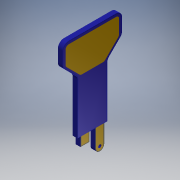
# Autodesk Inventor part: KeyerPaddle
Saved by Autodesk Inventor 2016 (Build 200138000, 138)
## iProperties
Created: 2016-06-11
Part Number: KeyerPaddle
Material: Generic
Document SubType Name: Modeling
Designer: Tyler
Density: 1 g/cm^3
Appearance: Default
Author: Tyler
Autodesk Inventor part; units mm, degrees
ref_plane "YZ Plane" through (0, 0, 0) normal (1, 0, 0) x (0, 1, 0)
ref_plane "XZ Plane" through (0, 0, 0) normal (0, 1, 0) x (-1, 0, 0)
ref_plane "XY Plane" through (0, 0, 0) normal (0, 0, 1) x (1, 0, 0)
sketch "Sketch1" plane through (0, 0, 0) normal (1, 0, 0) x (0, 1, 0)
  line L0 (0, 0) -> (1, 0)
  line L1 (1, 0) -> (1, -3)
  line L2 (1, -3) -> (4, -3)
  line L3 (4, -3) -> (4, 0)
  line L4 (4, 0) -> (5, 0)
  line L5 (5, 0) -> (5, 18)
  line L6 (5, 18) -> (10, 23)
  line L7 (10, 23) -> (10, 30)
  line L8 (10, 30) -> (0, 30)
  line L9 (0, 30) -> (0, 0)
  dimension "d0" = 1
  dimension "d1" = 3
  dimension "d2" = 1
  dimension "d3" = 3
  dimension "d4" = 30
  dimension "d5" = 7
  dimension "d6" = 45
  dimension "d7" = 10
  constraints: 20 end point, 6 parallel, 2 collinear, 1 horizontal, 1 perpendicular
  measures "d0" distance of L0.start L0.end
  measures "d1" distance of L1.end L2.end
  measures "d2" distance of L3.end L4.end
  measures "d3" distance between parallel lines of L4 L2
  measures "d4" distance from line of L4.end L8
  measures "d5" distance of L6.end L7.end
  measures "d6" angle of L5 L6
  measures "d7" distance between parallel lines of L9 L7
extrude "Extrusion1" add sketch "Sketch1" along normal blind 1.6
mirror "Mirror1" about plane through (0, 0, 30) normal (0, -1, 0) of "Extrusion1"
fillet "Fillet1" radius 2 6 edges at (0.8, 10, 30) (0.8, 10, 23) (0.8, -10, 30) (0.8, -10, 23) (0.8, -5, 18) (0.8, 5, 18)
sketch "Sketch2" plane through (1.6, 0, 0) normal (1, 0, 0) x (0, 0, -1)
  line L0 (0, 1) -> (3, 1) projected
  line L1 (3, 1) -> (3, 4) projected
  arc A0 (6, 1) -> (6, 4) centre (6, 2.5) ccw
  line L2 (3, 4) -> (6, 4)
  line L3 (3, 1) -> (6, 1)
  circle A1 centre (6, 2.5) radius 0.5
  point P0 (0, 0)
  dimension "d11" = 3
  dimension "d12" = 3
  dimension "d13" = 1
  constraints: 4 end point, 2 centre point, 2 point on circle, 2 tangent, 1 coincident, 1 collinear
  measures "d11" diameter of A0
  measures "d12" distance from line of A0.centre L1
  measures "d13" diameter of A1
extrude "Extrusion2" add sketch "Sketch2" against normal up to surface (1.6 mm away)
sketch "Sketch3" plane through (1.6, 0, 0) normal (1, 0, 0) x (0, 0, -1)
  line L0 (-30, 10) -> (7.5, 10) construction
  line L1 (7.5, 10) -> (7.5, -9.9928) construction
  line L2 (7.5, -9.9928) -> (-30, -9.9928) construction
  line L3 (-30, -9.9928) -> (-30, 10) construction
  line L4 (-23.8284, 10) -> (-28, 10) projected
  line L5 (-30, 8) -> (-30, -8) projected
  arc A0 (6, 1) -> (6, 4) centre (6, 2.5) ccw projected
  point P0 (0, 0)
  dimension "d17" = 1.5
  dimension "d18" = 1.5
  constraints: 2 collinear, 2 other
  measures "d17" distance from line of L1 A0.centre
  measures "d18" radius of A0
decal "Decal1"
sketch "Sketch4" plane through (0, 0, 0) normal (-1, 0, 0) x (0, 0, 1)
  line L0 (-7.5, 10) -> (30, 10) construction
  line L1 (30, 10) -> (30, -9.9928) construction
  line L2 (30, -9.9928) -> (-7.5, -9.9928) construction
  line L3 (-7.5, -9.9928) -> (-7.5, 10) construction
  line L4 (30, 8) -> (30, -8) projected
  line L5 (23.8284, 10) -> (28, 10) projected
  arc A0 (-6, 4) -> (-6, 1) centre (-6, 2.5) ccw projected
  point P0 (0, 0)
  dimension "d20" = 1.5
  constraints: 2 collinear, 2 other
  measures "d20" distance from line of L3 A0.centre
decal "Decal2"
equation "\"d17\" = d18"
equation "\"d20\" = d18"
body "Solid1"
